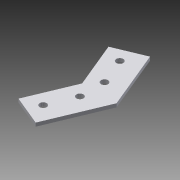
# Autodesk Inventor part: CornerBracket
Saved by Autodesk Inventor 2015 (Build 190159000, 159)
## iProperties
Created: 2015-01-26
Part Number: CornerBracket
Material: Aluminum 6061
Document SubType Name: Modeling
Designer: Andrew
Density: 2.7 g/cm^3
Appearance: Aluminum - Flat
CornerLength: 8.000 in
Author: Andrew
Autodesk Inventor part; units mm, degrees
ref_plane "YZ Plane" through (0, 0, 0) normal (1, 0, 0) x (0, 1, 0)
ref_plane "XZ Plane" through (0, 0, 0) normal (0, 1, 0) x (-1, 0, 0)
ref_plane "XY Plane" through (0, 0, 0) normal (0, 0, 1) x (1, 0, 0)
sketch "Sketch1" plane through (0, 0, 0) normal (0, 1, 0) x (-1, 0, 0)
  line L0 (0, 0) -> (21.3844, -51.6264)
  line L1 (21.3844, -51.6264) -> (47.9015, -40.6426)
  line L2 (47.9015, -40.6426) -> (31.0668, 0)
  line L3 (31.0668, 0) -> (47.9015, 40.6426)
  line L4 (47.9015, 40.6426) -> (21.3844, 51.6264)
  line L5 (21.3844, 51.6264) -> (0, 0)
  line L6 (31.0668, 0) -> (0, 0) construction
  line L7 (32.6076, 3.7198) -> (1.5408, 3.7198) construction
  line L8 (1.5408, -3.7198) -> (32.6076, -3.7198) construction
  line L9 (17.3204, 0) -> (53.6646, 87.7425) construction
  circle A0 centre (53.6646, 87.7425) radius 3.175 construction
  circle A1 centre (24.5041, -17.3428) radius 3.175
  circle A2 centre (34.2242, -40.8094) radius 3.175
  line L10 (31.0668, 0) -> (4.5496, 10.9838) construction
  circle A3 centre (43.9444, 64.2759) radius 3.175 construction
  circle A4 centre (34.2242, 40.8094) radius 3.175
  circle A5 centre (24.5041, 17.3428) radius 3.175
  line L11 (0, 0) -> (37.501, -15.5334) construction
  dimension "d1" = 55.88
  dimension "d2" = 135
  dimension "d3" = 3.7198
  dimension "d6" = 0
  dimension "d7" = 6.35
  dimension "d17" = 28.702
  dimension "d21" = 25.4
  dimension "d26" = 101.6
  dimension "d27" = 12.7
  constraints: 24 end point, 8 point on line, 6 centre point, 4 perpendicular, 3 parallel, 2 horizontal, 13 other
  measures "d1" distance of L4.end L0.start
  measures "d2" angle of L2 L3
  measures "d3" distance between parallel lines of L7 L6
  measures "d6" distance of A0.centre L9.end
  measures "d7" diameter of A0
  measures "d17" distance between parallel lines of L5 L3
  measures "d21" distance of A0.centre A3.centre
  measures "d26" distance from line of L9.end L11
  measures "d27" distance between parallel lines of L9 L3
extrude "Extrusion1" add sketch "Sketch1" along normal blind 3.175
equation "\"d26\" = 0.5 * CornerLength"
equation "\"d33\" = 0"
equation "\"CornerLength\" = 203.2"
body "Solid1"
